Autodesk Inventor part; units mm, degrees
(part 2 of 2)
sketch "Sketch14" plane through (0, 0, 0) normal (-1, 0, 0) x (0, 0, 1)
  line L0 (-11.7559, -167.3579) -> (7.4609, -167.3579) construction
  line L1 (7.4609, -167.3579) -> (7.4609, -166.0191) construction
  line L2 (7.4609, -166.0191) -> (-11.7559, -166.0191) construction
  line L3 (-11.7559, -166.0191) -> (-11.7559, -167.3579) construction
  line L4 (-24.7235, -175.3175) -> (-22.1546, -167.6975)
  line L5 (-22.1546, -167.6975) -> (-20.9073, -167.6975)
  line L6 (-20.9073, -167.6975) -> (-18.3385, -175.3175)
  line L7 (-18.3385, -175.3175) -> (-19.4067, -175.3175)
  line L8 (-19.4067, -175.3175) -> (-20.0984, -173.1871)
  line L9 (-20.0984, -173.1871) -> (-23.0068, -173.1871)
  line L10 (-23.0068, -173.1871) -> (-23.6984, -175.3175)
  line L11 (-23.6984, -175.3175) -> (-24.7235, -175.3175)
  line L12 (-20.3762, -172.3226) -> (-21.5557, -168.7349)
  line L13 (-21.5557, -168.7349) -> (-22.7289, -172.3226)
  line L14 (-22.7289, -172.3226) -> (-20.3762, -172.3226)
  line L15 (-11.7188, -175.3175) -> (-13.0341, -175.3175)
  line L16 (-13.0341, -175.3175) -> (-15.4424, -172.2855)
  line L17 (-15.4424, -172.2855) -> (-16.6033, -172.2855)
  line L18 (-16.6033, -172.2855) -> (-16.6033, -175.3175)
  line L19 (-16.6033, -175.3175) -> (-17.616, -175.3175)
  line L20 (-17.616, -175.3175) -> (-17.616, -167.6975)
  line L21 (-17.616, -167.6975) -> (-15.6523, -167.6975)
  spline S0 degree 2 poles (-15.6523, -167.6975) (-14.9978, -167.6975) (-14.1147, -167.8395) (-13.7134, -168.0989) knots 0 0 0 1 2 2 2
  spline S1 degree 2 poles (-13.7134, -168.0989) (-13.312, -168.3582) (-12.8489, -169.1671) (-12.8489, -169.7661) knots 0 0 0 1 2 2 2
  spline S2 degree 2 poles (-12.8489, -169.7661) (-12.8489, -170.5997) (-13.701, -171.7298) (-14.4297, -172.0015) knots 0 0 0 1 2 2 2
  line L22 (-14.4297, -172.0015) -> (-11.7188, -175.3175)
  spline S3 degree 2 poles (-13.9048, -169.8464) (-13.9048, -169.5129) (-14.1394, -169.0004) (-14.3864, -168.8337) knots 0 0 0 1 2 2 2
  spline S4 degree 2 poles (-14.3864, -168.8337) (-14.6026, -168.6917) (-15.1768, -168.5743) (-15.5967, -168.5743) knots 0 0 0 1 2 2 2
  line L23 (-15.5967, -168.5743) -> (-16.6033, -168.5743)
  line L24 (-16.6033, -168.5743) -> (-16.6033, -171.4396)
  line L25 (-16.6033, -171.4396) -> (-15.7141, -171.4396)
  spline S5 degree 2 poles (-15.7141, -171.4396) (-15.2756, -171.4396) (-14.5779, -171.2852) (-14.337, -171.0443) knots 0 0 0 1 2 2 2
  spline S6 degree 2 poles (-14.337, -171.0443) (-14.1147, -170.8344) (-13.9048, -170.2416) (-13.9048, -169.8464) knots 0 0 0 1 2 2 2
  line L26 (-9.3353, -175.3175) -> (-9.3353, -168.599)
  line L27 (-9.3353, -168.599) -> (-11.8917, -168.599)
  line L28 (-11.8917, -168.599) -> (-11.8917, -167.6975)
  line L29 (-11.8917, -167.6975) -> (-5.7661, -167.6975)
  line L30 (-5.7661, -167.6975) -> (-5.7661, -168.599)
  line L31 (-5.7661, -168.599) -> (-8.3226, -168.599)
  line L32 (-8.3226, -168.599) -> (-8.3226, -175.3175)
  line L33 (-8.3226, -175.3175) -> (-9.3353, -175.3175)
  spline S7 degree 2 poles (-2.87, -175.4533) (-3.6974, -175.4533) (-4.8584, -175.1075) (-5.3709, -174.8605) knots 0 0 0 1 2 2 2
  line L34 (-5.3709, -174.8605) -> (-5.3709, -173.5885)
  line L35 (-5.3709, -173.5885) -> (-5.2968, -173.5885)
  spline S8 degree 2 poles (-5.2968, -173.5885) (-4.7966, -174.0578) (-3.5307, -174.5765) (-2.9441, -174.5765) knots 0 0 0 1 2 2 2
  spline S9 degree 2 poles (-2.9441, -174.5765) (-2.1043, -174.5765) (-1.246, -173.8787) (-1.246, -173.3044) knots 0 0 0 1 2 2 2
  spline S10 degree 2 poles (-1.246, -173.3044) (-1.246, -172.8475) (-1.6967, -172.2794) (-2.1846, -172.1373) knots 0 0 0 1 2 2 2
  spline S11 degree 2 poles (-2.1846, -172.1373) (-2.5365, -172.0385) (-3.1232, -171.9027) (-3.5616, -171.7915) knots 0 0 0 1 2 2 2
  spline S12 degree 2 poles (-3.5616, -171.7915) (-3.9568, -171.6866) (-4.5805, -171.3716) (-4.8213, -171.1185) knots 0 0 0 1 2 2 2
  spline S13 degree 2 poles (-4.8213, -171.1185) (-5.056, -170.8653) (-5.3153, -170.186) (-5.3153, -169.7414) knots 0 0 0 1 2 2 2
  spline S14 degree 2 poles (-5.3153, -169.7414) (-5.3153, -168.8152) (-3.8703, -167.5616) (-2.7527, -167.5616) knots 0 0 0 1 2 2 2
  spline S15 degree 2 poles (-2.7527, -167.5616) (-2.1105, -167.5616) (-0.9743, -167.8148) (-0.4864, -168.0556) knots 0 0 0 1 2 2 2
  line L36 (-0.4864, -168.0556) -> (-0.4864, -169.2659)
  line L37 (-0.4864, -169.2659) -> (-0.5605, -169.2659)
  spline S16 degree 2 poles (-0.5605, -169.2659) (-0.9249, -168.9325) (-2.0611, -168.4385) (-2.6847, -168.4385) knots 0 0 0 1 2 2 2
  spline S17 degree 2 poles (-2.6847, -168.4385) (-3.3887, -168.4385) (-4.2594, -169.0992) (-4.2594, -169.6364) knots 0 0 0 1 2 2 2
  spline S18 degree 2 poles (-4.2594, -169.6364) (-4.2594, -170.1181) (-3.7468, -170.6924) (-3.2652, -170.822) knots 0 0 0 1 2 2 2
  spline S19 degree 2 poles (-3.2652, -170.822) (-2.9441, -170.9085) (-2.0117, -171.1308) (-1.7029, -171.2234) knots 0 0 0 1 2 2 2
  spline S20 degree 2 poles (-1.7029, -171.2234) (-0.9187, -171.4643) (-0.19, -172.4337) (-0.19, -173.1439) knots 0 0 0 1 2 2 2
  spline S21 degree 2 poles (-0.19, -173.1439) (-0.19, -173.5946) (-0.5544, -174.4591) (-0.8816, -174.7617) knots 0 0 0 1 2 2 2
  spline S22 degree 2 poles (-0.8816, -174.7617) (-1.246, -175.0952) (-2.1722, -175.4533) (-2.87, -175.4533) knots 0 0 0 1 2 2 2
  line L38 (3.4162, -172.4461) -> (0.5325, -172.4461)
  line L39 (0.5325, -172.4461) -> (0.5325, -171.5198)
  line L40 (0.5325, -171.5198) -> (3.4162, -171.5198)
  line L41 (3.4162, -171.5198) -> (3.4162, -172.4461)
  line L42 (9.0602, -175.3175) -> (4.645, -175.3175)
  line L43 (4.645, -175.3175) -> (4.645, -167.6975)
  line L44 (4.645, -167.6975) -> (5.6577, -167.6975)
  line L45 (5.6577, -167.6975) -> (5.6577, -174.4159)
  line L46 (5.6577, -174.4159) -> (9.0602, -174.4159)
  line L47 (9.0602, -174.4159) -> (9.0602, -175.3175)
  spline S23 degree 2 poles (12.969, -174.7123) (12.8517, -174.7988) (12.4565, -175.1075) (12.2712, -175.2002) knots 0 0 0 1 2 2 2
  spline S24 degree 2 poles (12.2712, -175.2002) (12.018, -175.336) (11.5426, -175.478) (11.1103, -175.478) knots 0 0 0 1 2 2 2
  spline S25 degree 2 poles (11.1103, -175.478) (10.7583, -175.478) (10.1223, -175.2125) (9.8815, -174.9717) knots 0 0 0 1 2 2 2
  spline S26 degree 2 poles (9.8815, -174.9717) (9.653, -174.737) (9.3751, -174.0454) (9.3751, -173.6626) knots 0 0 0 1 2 2 2
  spline S27 degree 2 poles (9.3751, -173.6626) (9.3751, -173.0698) (9.8753, -172.23) (10.4187, -171.9891) knots 0 0 0 1 2 2 2
  spline S28 degree 2 poles (10.4187, -171.9891) (10.9004, -171.7668) (12.2095, -171.6001) (12.969, -171.5569) knots 0 0 0 1 2 2 2
  line L48 (12.969, -171.5569) -> (12.969, -171.3716)
  spline S29 degree 2 poles (12.969, -171.3716) (12.969, -171.0382) (12.7652, -170.6244) (12.58, -170.5071) knots 0 0 0 1 2 2 2
  spline S30 degree 2 poles (12.58, -170.5071) (12.3947, -170.3898) (11.8637, -170.3157) (11.5796, -170.3157) knots 0 0 0 1 2 2 2
  spline S31 degree 2 poles (11.5796, -170.3157) (11.2462, -170.3157) (10.3446, -170.5133) (9.8938, -170.7047) knots 0 0 0 1 2 2 2
  line L49 (9.8938, -170.7047) -> (9.8382, -170.7047)
  line L50 (9.8382, -170.7047) -> (9.8382, -169.7229)
  spline S32 degree 2 poles (9.8382, -169.7229) (10.1038, -169.6488) (11.098, -169.4635) (11.5858, -169.4635) knots 0 0 0 1 2 2 2
  spline S33 degree 2 poles (11.5858, -169.4635) (12.1786, -169.4635) (12.9875, -169.6488) (13.3086, -169.8896) knots 0 0 0 1 2 2 2
  spline S34 degree 2 poles (13.3086, -169.8896) (13.6235, -170.1243) (13.9323, -170.8714) (13.9323, -171.4087) knots 0 0 0 1 2 2 2
  line L51 (13.9323, -171.4087) -> (13.9323, -175.3175)
  line L52 (13.9323, -175.3175) -> (12.969, -175.3175)
  line L53 (12.969, -175.3175) -> (12.969, -174.7123)
  line L54 (12.969, -173.9096) -> (12.969, -172.3226)
  spline S35 degree 2 poles (12.969, -172.3226) (12.6232, -172.3535) (11.5796, -172.4584) (11.2523, -172.5572) knots 0 0 0 1 2 2 2
  spline S36 degree 2 poles (11.2523, -172.5572) (10.8695, -172.6746) (10.3693, -173.1624) (10.3693, -173.5946) knots 0 0 0 1 2 2 2
  spline S37 degree 2 poles (10.3693, -173.5946) (10.3693, -174.0886) (10.9251, -174.5888) (11.4561, -174.5888) knots 0 0 0 1 2 2 2
  spline S38 degree 2 poles (11.4561, -174.5888) (11.9069, -174.5888) (12.6479, -174.1998) (12.969, -173.9096) knots 0 0 0 1 2 2 2
  spline S39 degree 2 poles (20.0765, -172.3658) (20.0765, -173.7675) (18.718, -175.478) (17.6929, -175.478) knots 0 0 0 1 2 2 2
  spline S40 degree 2 poles (17.6929, -175.478) (17.2298, -175.478) (16.569, -175.2496) (16.2479, -175.052) knots 0 0 0 1 2 2 2
  line L55 (16.2479, -175.052) -> (16.1862, -175.3175)
  line L56 (16.1862, -175.3175) -> (15.2846, -175.3175)
  line L57 (15.2846, -175.3175) -> (15.2846, -167.3579)
  line L58 (15.2846, -167.3579) -> (16.2479, -167.3579)
  line L59 (16.2479, -167.3579) -> (16.2479, -170.1984)
  spline S41 degree 2 poles (16.2479, -170.1984) (16.6123, -169.8711) (17.4582, -169.4388) (17.9955, -169.4388) knots 0 0 0 1 2 2 2
  spline S42 degree 2 poles (17.9955, -169.4388) (18.965, -169.4388) (20.0765, -170.9888) (20.0765, -172.3658) knots 0 0 0 1 2 2 2
  spline S43 degree 2 poles (19.0823, -172.4399) (19.0823, -171.4149) (18.4586, -170.3527) (17.767, -170.3527) knots 0 0 0 1 2 2 2
  spline S44 degree 2 poles (17.767, -170.3527) (17.378, -170.3527) (16.5752, -170.7232) (16.2479, -171.0073) knots 0 0 0 1 2 2 2
  line L60 (16.2479, -171.0073) -> (16.2479, -174.2862)
  spline S45 degree 2 poles (16.2479, -174.2862) (16.6123, -174.4653) (17.1742, -174.6135) (17.5076, -174.6135) knots 0 0 0 1 2 2 2
  spline S46 degree 2 poles (17.5076, -174.6135) (18.2425, -174.6135) (19.0823, -173.5699) (19.0823, -172.4399) knots 0 0 0 1 2 2 2
  point P0 (0, 0)
  constraints: 2 other
emboss "Emboss2" sketch "Sketch14" operation cut depth 2.54 direction (1, 0, 0)
sketch "Sketch15" plane through (0, -201.0841, 48.4212) normal (0, 0, 1) x (1, 0, 0)
  line L0 (21.59, 0) -> (21.59, 248.666) projected
  line L1 (17.272, 162.687) -> (21.59, 162.687)
  line L2 (21.59, 162.687) -> (21.59, 175.387)
  line L3 (21.59, 175.387) -> (17.272, 175.387)
  line L4 (17.272, 175.387) -> (17.272, 162.687)
  line L5 (21.59, 251.841) -> (0, 251.841) projected
  line L6 (0, -3.175) -> (21.59, -3.175) projected
  point P0 (0, 201.0841)
  point P1 (19.431, 175.387)
  dimension "d78" = 12.7
  dimension "d79" = 4.318
  dimension "d216" = 165.862
  constraints: 8 end point, 2 parallel, 1 horizontal, 1 midpoint, 1 perpendicular, 1 point on line
  measures "d78" distance of L3.end L1.start
  measures "d79" distance between parallel lines of L0 L4
  measures "d216" distance between parallel lines of L6 L1
extrude "Extrusion9" cut sketch "Sketch15" against normal blind 6.35
sketch "Sketch18" plane through (0, -204.2591, -52.5438) normal (0, -1, 0) x (1, 0, 0)
  line L0 (21.59, 45.8216) -> (21.59, 55.8292)
  line L1 (21.59, 55.8292) -> (20.3708, 55.8292)
  line L2 (20.3708, 55.8292) -> (18.6182, 53.8292)
  line L3 (18.6182, 47.8216) -> (18.6182, 53.8292)
  line L4 (21.59, 100.965) -> (0, 100.965) projected
  line L5 (21.59, 97.79) -> (21.59, 0) projected
  line L6 (21.59, 45.8216) -> (20.3708, 45.8216)
  line L7 (20.3708, 45.8216) -> (18.6182, 47.8216)
  point P0 (20.9804, 55.8292)
  dimension "d91" = 1.2192
  dimension "d92" = 2
  dimension "d94" = 6.0076
  dimension "d95" = 10.0076
  dimension "d98" = 1.7526
  dimension "d99" = 0
  dimension "d165" = 45.1358
  constraints: 12 end point, 1 horizontal, 1 midpoint
  measures "d91" distance of L0.end L1.end
  measures "d92" vertical distance of L1.end L2.end
  measures "d94" distance of L3.start L2.end
  measures "d95" distance of L0.start L0.end
  measures "d98" distance from line of L1.end L3
  measures "d99" distance between parallel lines of L5 L0
  measures "d165" distance from line of L4 point (20.98, 55.829)
extrude "Extrusion10" cut sketch "Sketch18" against normal blind 6.35
sketch "Sketch19" plane through (0, 13.9785, -4.7779) normal (-1, 0, 0) x (0, 0, 1)
  arc A0 (-43.686, 32.7145) -> (-46.7499, 29.4687) centre (-45.8609, 31.6985) ccw projected
  circle A1 centre (-45.8609, 31.6985) radius 4.5085
  arc A2 (45.9442, 32.7145) -> (49.0081, 29.4687) centre (48.1191, 31.6985) ccw projected
  circle A3 centre (48.1191, 31.6985) radius 4.5085
  circle A4 centre (-45.8609, -213.1575) radius 2.4005 projected
  circle A5 centre (-45.8609, -213.1575) radius 4.5085
  arc A6 (45.9433, -214.1716) -> (49.0081, -210.9277) centre (48.1191, -213.1575) ccw projected
  circle A7 centre (48.1191, -213.1575) radius 4.5085
  circle A8 centre (-41.4159, -64.8215) radius 4.5085
  circle A9 centre (-41.4159, -64.8215) radius 2.4005 projected
  circle A10 centre (43.6741, -64.8215) radius 4.5085
  circle A11 centre (43.6741, -64.8215) radius 2.4005 projected
  point P0 (0, 0)
  point P1 (48.9872, -224.0625)
  point P2 (-44.5909, 33.7355)
  point P3 (46.8491, 29.6614)
  point P4 (-48.0358, 32.7145)
  point P5 (45.9442, -204.0135)
  point P6 (49.0081, -200.7677)
  dimension "d110" = 9.017
  dimension "d111" = 9.017
  dimension "d112" = 9.017
  dimension "d113" = 9.017
  dimension "d120" = 9.017
  dimension "d121" = 0
  dimension "d122" = 0
  dimension "d123" = 9.017
  dimension "d124" = 0
  dimension "d125" = 0
  constraints: 6 centre point, 4 coincident
  measures "d110" diameter of A1
  measures "d111" diameter of A3
  measures "d112" diameter of A5
  measures "d113" diameter of A7
  measures "d120" diameter of A8
  measures "d121" distance of A9.centre A8.centre
  measures "d122" distance of A9.centre A8.centre
  measures "d123" diameter of A10
  measures "d124" distance of A11.centre A10.centre
  measures "d125" distance of A11.centre A10.centre
extrude "Extrusion11" cut sketch "Sketch19" against normal blind 5 contours A1 | A3 | A4 | A5 | A7 | A8 | A9 | A10 | A11
sketch "Sketch20" plane through (0, -204.2591, -52.5438) normal (0, -1, 0) x (1, 0, 0)
  circle A0 centre (19.558, 67.9574) radius 2.032
  line L0 (21.59, 100.965) -> (0, 100.965) projected
  line L1 (21.59, 97.79) -> (21.59, 55.8292) projected
  point P0 (0, 52.5438)
  dimension "d126" = 4.064
  dimension "d127" = 33.0076
  dimension "d128" = 2.032
  constraints: 1 centre point
  measures "d126" diameter of A0
  measures "d127" distance from line of L0 A0.centre
  measures "d128" distance from line of L1 A0.centre
extrude "Extrusion12" cut sketch "Sketch20" against normal blind 13.97
sketch "Sketch21" plane through (6.35, 0, 0) normal (1, 0, 0) x (0, 0, -1)
  line L0 (-35.2132, -45.6786) -> (-35.2132, -56.0144)
  line L1 (-42.0712, -70.6551) -> (-42.0712, -56.4311)
  line L2 (-36.9448, -42.8507) -> (-40.101, -41.2398)
  line L3 (-41.462, -39.9004) -> (-42.0712, -38.7527)
  line L4 (-36.9448, -58.8423) -> (-40.101, -60.4532)
  line L5 (-41.462, -61.7925) -> (-42.0712, -62.9403)
  arc A0 (-41.462, -39.9004) -> (-40.101, -41.2398) centre (-38.6576, -38.4118) ccw
  arc A1 (-40.101, -60.4532) -> (-41.462, -61.7925) centre (-38.6576, -63.2812) ccw
  arc A2 (-36.9448, -58.8423) -> (-35.2132, -56.0144) centre (-38.3882, -56.0144) ccw
  arc A3 (-35.2132, -45.6786) -> (-36.9448, -42.8507) centre (-38.3882, -45.6786) ccw
  line L6 (46.8288, -56.4311) -> (46.8288, -70.6551)
  line L7 (42.5108, -56.0234) -> (42.5108, -45.6876)
  line L8 (44.2424, -42.8597) -> (47.392, -41.2521)
  line L9 (48.753, -39.9128) -> (49.3688, -38.7527)
  line L10 (44.2424, -58.8513) -> (47.392, -60.4589)
  line L11 (48.753, -61.7982) -> (49.3688, -62.9583)
  arc A4 (48.753, -61.7982) -> (47.392, -60.4589) centre (45.9486, -63.2868) ccw
  arc A5 (42.5108, -56.0234) -> (44.2424, -58.8513) centre (45.6858, -56.0234) ccw
  arc A6 (47.392, -41.2521) -> (48.753, -39.9128) centre (45.9486, -38.4241) ccw
  arc A7 (44.2424, -42.8597) -> (42.5108, -45.6876) centre (45.6858, -45.6876) ccw
  line L12 (49.3688, -38.7527) -> (49.3688, -62.9583)
  line L13 (-42.0712, -38.7527) -> (-42.0712, -62.9403)
  line L14 (49.3688, -38.7527) -> (49.3688, -62.9583)
  line L15 (49.3688, -194.7341) -> (49.3688, 41.2319) projected
  circle A8 centre (-38.8962, -50.8431) radius 2.4005 projected
  circle A9 centre (-38.8962, -50.8431) radius 2.4005
  line L16 (49.3688, 41.2319) -> (49.3688, -194.7341) projected
  line L17 (49.3688, -38.7527) -> (49.3688, -62.9583)
  circle A10 centre (46.1938, -50.8431) radius 2.4005 projected
  circle A11 centre (46.1938, -50.8431) radius 2.4005
  point P0 (0, 0)
  point P1 (-37.8414, -63.5431)
  point P2 (-37.853, -70.6551)
  point P3 (-37.853, -56.4311)
  point P4 (-40.9926, -40.7847)
  point P5 (-40.9926, -60.9083)
  point P6 (43.3998, -52.8751)
  point P7 (48.2836, -40.797)
  point P8 (46.8288, -57.8659)
  point P9 (46.8288, -56.4311)
  point P10 (46.8288, -57.8659)
  point P11 (-42.0712, -62.9403)
  point P12 (46.8288, -43.726)
  point P13 (46.8288, -47.8001)
  point P14 (49.3688, 43.6399)
  point P15 (49.3688, 50.7569)
  dimension "d135" = 14.224
  dimension "d168" = 145
  dimension "d169" = 145
  dimension "d170" = 117.04
  dimension "d171" = 117.04
  dimension "d172" = 2.032
  dimension "d173" = 2.032
  dimension "d175" = 3.175
  dimension "d176" = 3.1561
  dimension "d177" = 3.1561
  dimension "d181" = 145
  dimension "d182" = 145
  dimension "d183" = 117.04
  dimension "d184" = 117.04
  dimension "d185" = 3.175
  dimension "d187" = 3.175
  dimension "d188" = 3.1496
  dimension "d189" = 2.0443
  dimension "d190" = 3.1496
  dimension "d204" = 24.1877
  dimension "d209" = 24.2056
  dimension "d215" = 0
  dimension "d218" = 12.0904
  dimension "d219" = 12.0904
  constraints: 30 end point, 16 point on circle, 16 tangent, 10 centre point, 8 point on line, 7 equal radius, 2 coincident, 2 parallel, 2 vertical, 3 other
  measures "d135" distance of point (-37.853, -70.655) point (-37.853, -56.431)
  measures "d168" angle of L2 L3
  measures "d169" angle of L5 L4
  measures "d170" angle of L4 L0
  measures "d171" angle of L0 L2
  measures "d172" vertical distance of point (-40.993, -40.785) L3.end
  measures "d173" vertical distance of point (-40.993, -60.908) L5.end
  measures "d175" radius of A0
  measures "d176" horizontal distance of L2.start L2.end
  measures "d177" horizontal distance of L4.start L4.end
  measures "d181" angle of L8 L9
  measures "d182" angle of L11 L10
  measures "d183" angle of L10 L7
  measures "d184" angle of L7 L8
  measures "d185" radius of A4
  measures "d187" radius of A6
  measures "d188" horizontal distance of L8.start L8.end
  measures "d189" vertical distance of L9.end point (48.284, -40.797)
  measures "d190" horizontal distance of L10.start L10.end
  measures "d204" distance of L5.end L3.end
  measures "d209" distance of L11.end L9.end
  measures "d215" horizontal extent of L15
  measures "d218" vertical distance of A8.centre L3.end
  measures "d219" vertical distance of A10.centre L17.start
extrude "Extrusion13" add sketch "Sketch21" along normal blind 10.16
sketch "Sketch22" plane through (0, -204.2591, -52.5438) normal (0, -1, 0) x (1, 0, 0)
  line L0 (21.59, 67.9574) -> (21.59, 45.8216) projected
  line L1 (13.97, 9.525) -> (21.59, 9.525)
  line L2 (21.59, 9.525) -> (21.59, 88.265)
  line L3 (21.59, 88.265) -> (13.97, 88.265)
  line L4 (13.97, 88.265) -> (13.97, 9.525)
  line L5 (21.59, 100.965) -> (0, 100.965) projected
  line L6 (0, -3.175) -> (21.59, -3.175) projected
  line L7 (10.4902, 45.3136) -> (13.97, 45.3136)
  line L8 (13.97, 45.3136) -> (13.97, 56.3372)
  line L9 (13.97, 56.3372) -> (10.4902, 56.3372)
  line L10 (10.4902, 56.3372) -> (10.4902, 45.3136)
  line L11 (21.59, 56.3372) -> (20.1405, 56.3372) projected
  line L12 (20.1405, 45.3136) -> (21.59, 45.3136) projected
  line L13 (18.1102, 54.0203) -> (18.1102, 47.6305) projected
  point P0 (0, 52.5438)
  point P1 (21.59, 93.599)
  point P2 (17.78, 88.265)
  point P3 (17.78, 9.525)
  point P4 (20.8653, 56.3372)
  point P5 (12.2301, 56.3372)
  point P6 (20.8653, 45.3136)
  point P7 (10.4902, 50.8254)
  dimension "d191" = 12.7
  dimension "d192" = 12.7
  dimension "d193" = 0
  dimension "d194" = 0
  dimension "d195" = 7.62
  dimension "d203" = 7.62
  constraints: 16 end point, 6 midpoint, 4 parallel, 2 horizontal, 2 perpendicular, 2 point on line
  measures "d191" distance from line of L5 point (17.78, 88.265)
  measures "d192" distance from line of L6 point (17.78, 9.525)
  measures "d193" vertical distance of point (20.865, 56.337) point (12.23, 56.337)
  measures "d194" distance from line of point (20.865, 45.314) L7
  measures "d195" distance from line of L13 point (10.49, 50.825)
  measures "d203" distance between parallel lines of L2 L4
extrude "Extrusion14" cut sketch "Sketch22" against normal blind 7.62
fillet "Fillet7" radius 0.762 4 edges at (10.4902, -201.0841, 3.7934) (10.4902, -201.0841, -7.2302) (13.97, -201.0841, -7.2302) (13.97, -201.0841, 3.7934)
fillet "Fillet8" radius 0.762 11 edges at (13.7468, -204.2591, 4.0166) (12.2301, -204.2591, 3.7934) (10.7134, -204.2591, 3.5702) (10.4902, -204.2591, -1.7184) (10.7134, -204.2591, -7.007) (12.2301, -204.2591, -7.2302) (13.7468, -204.2591, -7.4534) (13.97, -204.2591, -25.5055) (13.97, -204.2591, 20.1383) (17.78, -204.2591, -43.0188) (17.78, -204.2591, 35.7212)
sketch "Sketch23" plane through (17.78, 46.6929, 14.1312) normal (1, 0, 0) x (0, 0, -1)
  line L0 (0, 4.064) -> (57.15, 4.064) projected
  line L1 (0, 0) -> (57.15, 0) projected
  line L2 (57.15, 4.064) -> (38.1, 4.064)
  line L3 (38.1, 4.064) -> (38.1, 0)
  line L4 (38.1, 0) -> (57.15, 0)
  line L5 (57.15, 0) -> (57.15, 4.064)
  line L6 (0, 0) -> (0, 4.064) projected
  point P0 (14.1312, -46.6929)
  point P1 (0, 2.032)
  point P2 (38.1, 4.064)
  dimension "d221" = 38.1
  constraints: 8 end point, 2 parallel, 1 horizontal, 1 midpoint, 1 perpendicular, 1 point on line
  measures "d221" distance from line of point (0, 2.032) L3
extrude "Extrusion15" add sketch "Sketch23" along normal blind 10.16 contours L0 L5 L1 L3
fillet "Fillet9" radius 0.508 5 edges at (19.685, 50.7569, 14.1312) (17.78, 50.7569, -4.9188) (22.86, 50.7569, -23.9688) (27.94, 50.7569, -33.4938) (24.765, 50.7569, -43.0188)
body "Solid1"
